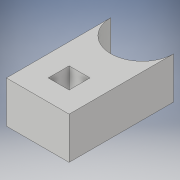
# Autodesk Inventor part: Part27
Saved by Autodesk Inventor 2019 (Build 230136000, 136)
## iProperties
Created: 2021-08-31
Part Number: Part27
Material: 一般
Document SubType Name: Sheet Metal
Designer: yuta
Density: 1 g/cm^3
Sheet Metal Rule: Default_mm
Appearance: 既定
Author: yuta
Autodesk Inventor part; units mm, degrees
ref_plane "YZ Plane" through (0, 0, 0) normal (1, 0, 0) x (0, 1, 0)
ref_plane "XZ Plane" through (0, 0, 0) normal (0, 1, 0) x (-1, 0, 0)
ref_plane "XY Plane" through (0, 0, 0) normal (0, 0, 1) x (1, 0, 0)
sketch "スケッチ1" plane through (0, 0, 0) normal (0, 1, 0) x (-1, 0, 0)
  line L0 (8.4764, 10.991) -> (-21.5236, 10.991)
  line L1 (-21.5236, 10.991) -> (-21.5236, -39.009)
  line L2 (-21.5236, -39.009) -> (8.4764, -39.009)
  line L3 (8.4764, -39.009) -> (8.4764, 10.991)
  point P0 (0, 0)
  dimension "d0" = 30
  dimension "d1" = 50
  constraints: 8 end point, 2 parallel, 1 horizontal, 1 perpendicular
  measures "d0" distance of L2.end L1.end
  measures "d1" distance of L1.end L0.end
extrude "押し出し1" add sketch "スケッチ1" along normal blind 20
sketch "スケッチ2" plane through (0, 20, 0) normal (0, 1, 0) x (1, 0, 0)
  line L0 (21.5236, 39.009) -> (-8.4764, 39.009) projected
  circle A0 centre (6.5236, 39.009) radius 15
  point P0 (0, 0)
  dimension "d4" = 30
  constraints: 1 centre point, 1 midpoint
  measures "d4" diameter of A0
hole "穴1" at (6.5236, 20, -39.009) direction (0, -1, 0) diameter 30 depth 20
sketch "スケッチ3" plane through (0, 20, 0) normal (0, 1, 0) x (1, 0, 0)
  line L0 (1.5236, -0.991) -> (11.5236, -0.991)
  line L1 (11.5236, -0.991) -> (11.5236, 9.009)
  line L2 (11.5236, 9.009) -> (1.5236, 9.009)
  line L3 (1.5236, 9.009) -> (1.5236, -0.991)
  line L4 (-8.4764, 39.009) -> (-8.4764, -10.991) projected
  line L5 (-8.4764, -10.991) -> (21.5236, -10.991) projected
  point P0 (0, 0)
  dimension "d12" = 10
  dimension "d13" = 10
  dimension "d14" = 10
  dimension "d15" = 10
  constraints: 8 end point, 2 parallel, 1 horizontal, 1 perpendicular
  measures "d12" distance of L2.end L1.end
  measures "d13" distance of L1.end L0.end
  measures "d14" distance between parallel lines of L3 L4
  measures "d15" distance between parallel lines of L5 L0
extrude "押し出し2" cut sketch "スケッチ3" against normal blind 20
equation "\"BendRadius\" = Thickness"
equation "\"BendReliefWidth\" = Thickness"
equation "\"BendReliefDepth\" = 0.5 * Thickness"
equation "\"CornerReliefSize\" = 4 * Thickness"
equation "\"MinimumRemnant\" = 2 * Thickness"
equation "\"TransitionRadius\" = BendRadius"
equation "\"JacobiRadiusSize\" = BendRadius"
equation "\"GapSize\" = Thickness"
equation "\"Thickness\" = 0.5"
